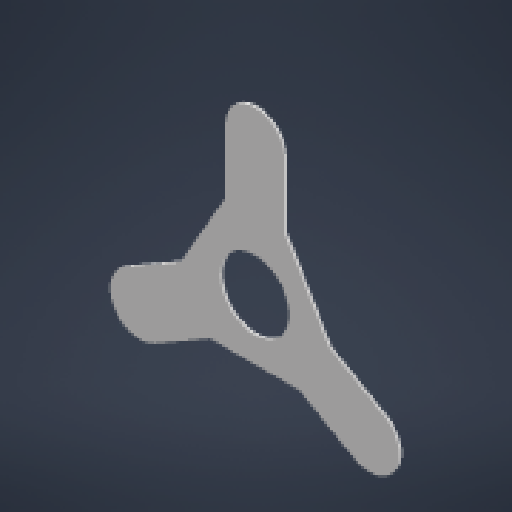
# Autodesk Inventor part: Bund
Saved by Autodesk Inventor 2026.1 (Build 301233020, 233B)
## iProperties
Created: 2025-11-07
Part Number: Bund
Material: Generic
Document SubType Name: Modeling
Designer: Mikke
Density: 1 g/cm^3
Appearance: Default
Author: Mikke
Autodesk Inventor part; units mm, degrees
ref_plane "YZ Plane" through (0, 0, 0) normal (1, 0, 0) x (0, 1, 0)
ref_plane "XZ Plane" through (0, 0, 0) normal (0, 1, 0) x (-1, 0, 0)
ref_plane "XY Plane" through (0, 0, 0) normal (0, 0, 1) x (1, 0, 0)
ref_plane "Work Plane1" through (0, 0, 0) normal (0, 0, 1) x (1, 0, 0)
sketch "Sketch1" plane through (0, 0, 0) normal (0, 0, 1) x (1, 0, 0)
  circle A0 centre (25, -136.9573) radius 110
  line L0 (-96.6901, -226.845) -> (-113.6901, -197.4001)
  line L1 (-100.9544, -229.307) -> (-117.9544, -199.8621)
  line L2 (163.6901, -197.4001) -> (146.6901, -226.845)
  line L3 (167.9544, -199.8621) -> (150.9544, -229.307)
  line L4 (8, 13.3733) -> (42, 13.3733)
  line L5 (8, 18.2974) -> (42, 18.2974)
  line L6 (25, -136.9573) -> (25, 18.2974)
  line L7 (25, -136.9573) -> (159.4544, -214.5846)
  line L8 (25, -136.9573) -> (-109.4544, -214.5846)
  line L9 (-10, -136.9573) -> (-10, 18.2974)
  line L10 (60, -136.9573) -> (60, 18.2974)
  line L11 (42.5, -106.6464) -> (176.9544, -184.2737)
  line L12 (7.5, -167.2681) -> (141.9544, -244.8954)
  line L13 (42.5, -167.2681) -> (-91.9544, -244.8954)
  line L14 (7.5, -106.6464) -> (-126.9544, -184.2737)
  arc A1 (141.9544, -244.8954) -> (176.9544, -184.2737) centre (159.4544, -214.5846) ccw
  arc A2 (60, 18.2974) -> (-10, 18.2974) centre (25, 18.2974) ccw
  arc A3 (-126.9544, -184.2737) -> (-91.9544, -244.8954) centre (-109.4544, -214.5846) ccw
  line L15 (25, -177.3718) -> (76.9615, -207.3718)
  line L16 (-10, -116.75) -> (-61.9615, -146.75)
  line L17 (-10, -116.75) -> (-10, -56.75)
  line L18 (60, -116.75) -> (60, -56.75)
  line L19 (60, -116.75) -> (111.9615, -146.75)
  line L20 (111.9615, -146.75) -> (60, -56.75)
  line L21 (-10, -56.75) -> (-61.9615, -146.75)
  line L22 (25, -177.3718) -> (-26.9615, -207.3718)
  line L23 (-26.9615, -207.3718) -> (76.9615, -207.3718)
  circle A4 centre (25, -136.9573) radius 40.4145
  point P0 (0, 0)
extrude "Extrusion1" add sketch "Sketch1" along normal blind 3 contours L10 A4 L6 A0 | A0 L9 A2 L10 | L11 A1 L12 A0 | A0 L7 A4 L11 | L6 A4 L9 A0 | L20 L11 L10 | A0 L12 A4 L7 | L14 A4 L8 A0 | A0 L13 A3 L14 | L9 L14 L21 | A0 L8 A4 L13 | L23 L13 L12
sketch "Sketch3" plane through (0, 0, 0) normal (0, 0, -1) x (-1, 0, 0)
  circle A0 centre (-40, -1.2646) radius 1.5 projected
  circle A1 centre (-10, -1.2646) radius 1.5 projected
  circle A2 centre (-10, 31.4848) radius 1.5 projected
  circle A3 centre (-40, 31.4848) radius 1.5 projected
  circle A4 centre (113.3751, -234.1687) radius 1.5 projected
  circle A5 centre (85.0133, -217.794) radius 1.5 projected
  circle A6 centre (100.0133, -191.8132) radius 1.5 projected
  circle A7 centre (128.3751, -208.1879) radius 1.5 projected
  circle A8 centre (-135.0133, -217.794) radius 1.5 projected
  circle A9 centre (-163.3751, -234.1687) radius 1.5 projected
  circle A10 centre (-178.3751, -208.1879) radius 1.5 projected
  circle A11 centre (-150.0133, -191.8132) radius 1.5 projected
  point P0 (0, 0)
extrude "Extrusion2" cut sketch "Sketch3" against normal blind 6
body "Solid1"
